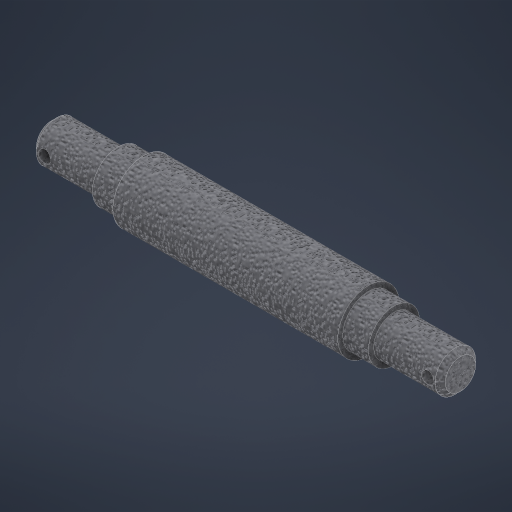
# Autodesk Inventor part: Axel
Saved by Autodesk Inventor 2024.1 (Build 281209000, 209)
## iProperties
Created: 2023-10-20
Part Number: Axel
Material: Iron, Cast
Document SubType Name: Modeling
Designer: LEGION SMIT
Density: 7.15 g/cm^3
Appearance: Iron - Cast
Author: LEGION SMIT
Autodesk Inventor part; units mm, degrees
ref_plane "YZ Plane" through (0, 0, 0) normal (1, 0, 0) x (0, 1, 0)
ref_plane "XZ Plane" through (0, 0, 0) normal (0, 1, 0) x (-1, 0, 0)
ref_plane "XY Plane" through (0, 0, 0) normal (0, 0, 1) x (1, 0, 0)
sketch "Sketch1" plane through (0, 0, 0) normal (0, 1, 0) x (-1, 0, 0)
  line L0 (0, 0) -> (80, 0)
  line L1 (80, 0) -> (80, 3.95)
  line L2 (80, 3.95) -> (67, 3.95)
  line L3 (67, 3.95) -> (67, 5)
  line L4 (67, 5) -> (62, 5)
  line L5 (62, 5) -> (62, 6)
  line L6 (62, 6) -> (18, 6)
  line L7 (18, 6) -> (18, 5)
  line L8 (18, 5) -> (13, 5)
  line L9 (13, 5) -> (13, 3.95)
  line L10 (13, 3.95) -> (0, 3.95)
  line L11 (0, 3.95) -> (0, 0)
  point P0 (40, 6)
  dimension "d0" = 80
  dimension "d1" = 3.95
  dimension "d2" = 18
  dimension "d3" = 5
  dimension "d4" = 5
  dimension "d5" = 6
  dimension "d6" = 22
  dimension "d7" = 5
  constraints: 24 end point, 9 perpendicular, 4 point on line, 1 horizontal, 1 midpoint
  measures "d0" distance of L0.start L0.end
  measures "d1" distance of L0.end L1.end
  measures "d2" distance from line of L4.end L1
  measures "d3" distance of L3.end L4.end
  measures "d4" distance between parallel lines of L0 L4
  measures "d5" distance between parallel lines of L0 L6
  measures "d6" distance of L5.end point (40, 6)
  measures "d7" distance of L7.end L8.end
revolve "Revolution1" add sketch "Sketch1" angle 360 about axis through (0, 0, 0) along (-1, 0, 0)
chamfer "Chamfer1" distance 1 angle 45 2 edges at (-80, 0, -3.95) (0, 0, -3.95)
sketch "Sketch2" plane through (0, 0, 0) normal (0, 1, 0) x (-1, 0, 0)
  circle A0 centre (77.5, 0) radius 1.2
  line L0 (80, 2.95) -> (80, -2.95) projected
  circle A1 centre (2.5, 0) radius 1.2
  line L1 (0, -2.95) -> (0, 2.95) projected
  point P0 (0, 0)
  dimension "d12" = 2.4
  dimension "d13" = 2.5
  dimension "d14" = 2.4
  dimension "d15" = 2.5
  constraints: 2 centre point
  measures "d12" diameter of A0
  measures "d13" distance from line of L0 A0.centre
  measures "d14" diameter of A1
  measures "d15" distance from line of L1 A1.centre
extrude "Extrusion1" cut sketch "Sketch2" along normal mid plane 10
body "Solid1"
